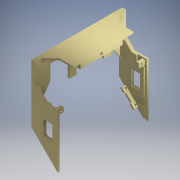
# Autodesk Inventor part: obudowa
Saved by Autodesk Inventor 2017 (Build 210142000, 142)
## iProperties
Created: 2016-11-10
Part Number: obudowa
Material: Generic
Document SubType Name: Modeling
Designer: Shichi
Density: 1 g/cm^3
Appearance: Gold - Metal
Author: Shichi
Autodesk Inventor part; units mm, degrees
ref_plane "YZ Plane" through (0, 0, 0) normal (1, 0, 0) x (0, 1, 0)
ref_plane "XZ Plane" through (0, 0, 0) normal (0, 1, 0) x (-1, 0, 0)
ref_plane "XY Plane" through (0, 0, 0) normal (0, 0, 1) x (1, 0, 0)
sketch "Sketch1" plane through (0, 0, 0) normal (0, 1, 0) x (-1, 0, 0)
  line L0 (0, 0) -> (29, 0)
  line L1 (29, 0) -> (29, 64)
  line L2 (29, 64) -> (25, 64)
  line L3 (25, 64) -> (25, 30)
  line L4 (25, 30) -> (0, 30)
  line L5 (0, 30) -> (0, 0)
  line L6 (29, 0) -> (0, -29)
  line L7 (0, 0) -> (0, -29)
  dimension "d0" = 29
  dimension "d1" = 64
  dimension "d2" = 4
  dimension "d47" = 34
  dimension "d48" = 45
  constraints: 16 end point, 5 perpendicular, 1 horizontal, 1 vertical
  measures "d0" distance of L0.start L0.end
  measures "d1" distance of L0.end L1.end
  measures "d2" distance of L1.end L2.end
  measures "d47" distance of L2.end L3.end
  measures "d48" angle of L6 L0
extrude "Extrusion1" add sketch "Sketch1" along normal blind 2
sketch "Sketch4" plane through (-29, 0, 64) normal (0, 0, 1) x (1, 0, 0)
  line L0 (29, 2) -> (0, 2) projected
  line L1 (0, 2) -> (0, 50)
  line L2 (4, 0) -> (4, 2) projected
  line L3 (4, 2) -> (4, 17)
  line L4 (4, 17) -> (29, 17)
  line L5 (29, 17) -> (29, 50)
  line L6 (0, 50) -> (29, 50)
  point P0 (29, 0)
  dimension "d6" = 48
  dimension "d7" = 15
  dimension "d8" = 25
  dimension "d9" = 33
  constraints: 10 end point, 2 vertical alignment, 1 horizontal, 1 vertical
  measures "d6" distance of L0.end L1.end
  measures "d7" distance of L2.end L3.end
  measures "d8" distance of L3.end L4.end
  measures "d9" distance of L4.end L5.end
extrude "Extrusion2" add sketch "Sketch4" against normal blind 2
ref_plane "Work Plane1" through (0, 50, 0) normal (0, 1, 0) x (1, 0, 0)
mirror "Mirror2" about plane through (0, 50, 0) normal (0, 1, 0) of "Extrusion1"
mirror "Mirror1" about plane through (-29, 50, 64) normal (0, 1, 0) of "Extrusion2"
sketch "Sketch6" plane through (-29, 0, 0) normal (-1, 0, 0) x (0, 0, 1)
  line L0 (62, 17) -> (62, 83) projected
  line L1 (62, 66) -> (16.2993, 98)
  line L2 (62, 98) -> (30, 98) projected
  line L3 (62, 98) -> (62, 66)
  line L4 (16.2993, 98) -> (62, 98)
  point P0 (0, 0)
  dimension "d13" = 32
  dimension "d14" = 55
  constraints: 6 end point, 2 point on line, 1 collinear, 1 vertical
  measures "d13" distance of L2.start L1.start
  measures "d14" angle of L1 L3
extrude "Extrusion3" add sketch "Sketch6" against normal blind 4
sketch "Sketch8" plane through (0, 0, 30) normal (1, 0, 0) x (0, 0, -1)
  line L0 (0, 0) -> (0, 2) projected
  line L1 (0, 2) -> (59, 2) projected
  line L2 (1.5, 2) -> (6.5, 2)
  line L3 (6.5, 2) -> (6.5, 8.5)
  line L4 (6.5, 8.5) -> (1.5, 8.5)
  line L5 (1.5, 8.5) -> (1.5, 2)
  line L6 (-32, 2) -> (0, 2) construction
  line L7 (0, 2) -> (0, 17.9945) construction
  circle A0 centre (4, 6) radius 1.25
  point P0 (30, 0)
  point P1 (30, 2)
  dimension "d17" = 6.5
  dimension "d18" = 6.5
  dimension "d22" = 1.5
  dimension "d23" = 2.5
  dimension "d24" = 4
  dimension "d25" = 4
  constraints: 10 end point, 2 horizontal alignment, 2 parallel, 1 centre point, 1 horizontal, 1 perpendicular, 1 point on line, 1 vertical, 1 vertical alignment
  measures "d17" distance of L4.end L2.start
  measures "d18" distance between parallel lines of L3 L7
  measures "d22" distance between parallel lines of L7 L5
  measures "d23" diameter of A0
  measures "d24" horizontal distance of L0.end A0.centre
  measures "d25" distance from line of A0.centre L1
extrude "Extrusion4" add sketch "Sketch8" against normal blind 5
sketch "Sketch9" plane through (0, 17, 64) normal (1, 0, 0) x (0, 0, -1)
  circle A0 centre (5.7, 33) radius 1.25
  line L0 (2, 0) -> (2, 66) projected
  line L1 (0, 66) -> (2, 66) projected
  line L2 (2, 36.25) -> (8.95, 36.25)
  line L3 (8.95, 36.25) -> (8.95, 29.75)
  line L4 (8.95, 29.75) -> (2, 29.75)
  line L5 (2, 29.75) -> (2, 36.25)
  line L6 (5.7, 34.25) -> (7.6582, 34.25) construction
  line L7 (6.95, 33) -> (6.95, 31.8854) construction
  point P0 (64, -17)
  dimension "d28" = 2.5
  dimension "d29" = 3.7
  dimension "d30" = 33
  dimension "d32" = 2
  dimension "d33" = 4.5
  dimension "d34" = 2
  constraints: 12 end point, 2 horizontal, 2 parallel, 2 point on circle, 2 tangent, 1 centre point, 1 perpendicular, 1 point on line, 1 vertical
  measures "d28" diameter of A0
  measures "d29" distance from line of L0 A0.centre
  measures "d30" distance from line of A0.centre L1
  measures "d32" distance between parallel lines of L2 L6
  measures "d33" distance between parallel lines of L4 L6
  measures "d34" distance between parallel lines of L3 L7
extrude "Extrusion5" add sketch "Sketch9" against normal blind 5
extrude "Extrusion6" cut sketch "Sketch8" against normal blind 2
mirror "Mirror3" about plane through (0, 50, 0) normal (0, 1, 0) of "Extrusion3", "Extrusion4", "Extrusion6"
extrude "Extrusion7" cut sketch "Sketch9" against normal blind 2
sketch "Sketch10" plane through (-29, 0, 62) normal (0, 0, -1) x (-1, 0, 0)
  line L0 (-15, 27) -> (-13, 27)
  line L1 (-13, 27) -> (-13, 35)
  line L2 (-13, 35) -> (-15, 35)
  line L3 (-15, 35) -> (-15, 27)
  line L4 (-24, 53.25) -> (-24, 46.75) projected
  line L5 (-29, 17) -> (-4, 17) projected
  line L6 (-29, 17) -> (-29, 83) construction
  line L7 (-29, 50) -> (0, 50) construction
  line L8 (0, 34) -> (0, 66) construction
  line L9 (-15, 73) -> (-13, 73)
  line L10 (-13, 73) -> (-13, 65)
  line L11 (-13, 65) -> (-15, 65)
  line L12 (-15, 65) -> (-15, 73)
  point P0 (-29, 0)
  point P1 (-15, 31)
  dimension "d41" = 9
  dimension "d42" = 2
  dimension "d43" = 8
  dimension "d46" = 10
  constraints: 18 end point, 4 symmetric about line, 3 midpoint, 2 parallel, 1 horizontal, 1 perpendicular
  measures "d41" distance between parallel lines of L4 L3
  measures "d42" distance of L0.start L0.end
  measures "d43" distance of L0.end L1.end
  measures "d46" distance from line of L5 L0.end
extrude "Extrusion8" add sketch "Sketch10" along normal blind 22
sketch "Sketch11" plane through (-25, 100, 30) normal (0, 1, 0) x (1, 0, 0)
  line L0 (9, 16) -> (19, 16)
  line L1 (19, 16) -> (19, 33)
  line L2 (19, 33) -> (9, 33)
  line L3 (9, 33) -> (9, 16)
  line L4 (0, 0) -> (25, 0) projected
  line L5 (25, 0) -> (25, 59) projected
  point P0 (25, 30)
  dimension "d49" = 16
  dimension "d50" = 6
  dimension "d51" = 10
  dimension "d52" = 17
  constraints: 8 end point, 2 parallel, 1 horizontal, 1 horizontal alignment, 1 perpendicular
  measures "d49" distance between parallel lines of L4 L0
  measures "d50" distance between parallel lines of L5 L1
  measures "d51" distance of L1.end L2.end
  measures "d52" distance of L0.end L1.end
extrude "Extrusion9" cut sketch "Sketch11" against normal through all
sketch "Sketch12" plane through (-29, 0, 0) normal (-0.7071068, 0, -0.7071068) x (-0.7071068, 0, 0.7071068)
  line L0 (0.7071, 2) -> (-41.0122, 2) projected
  line L1 (-8, 2) -> (-13, 2)
  line L2 (-13, 2) -> (-13, 8)
  line L3 (-13, 8) -> (-8, 8)
  line L4 (-8, 8) -> (-8, 2)
  line L5 (-23, 2) -> (-28, 2)
  line L6 (-28, 2) -> (-28, 8)
  line L7 (-28, 8) -> (-23, 8)
  line L8 (-23, 8) -> (-23, 2)
  line L9 (0, 0) -> (0, 2) projected
  circle A0 centre (-10.5, 5) radius 1.25
  circle A1 centre (-25.5, 5) radius 1.25
  point P0 (-20.5061, 0)
  dimension "d55" = 8
  dimension "d56" = 5
  dimension "d57" = 6
  dimension "d58" = 10
  dimension "d59" = 5
  dimension "d60" = 6
  dimension "d61" = 2.5
  dimension "d62" = 2.5
  dimension "d63" = 3
  dimension "d64" = 2.5
  dimension "d65" = 3
  dimension "d66" = 2.5
  constraints: 16 end point, 4 parallel, 2 centre point, 2 horizontal, 2 perpendicular, 2 point on line
  measures "d55" distance between parallel lines of L4 L9
  measures "d56" distance of L2.end L3.end
  measures "d57" distance of L1.end L2.end
  measures "d58" distance between parallel lines of L2 L8
  measures "d59" distance of L6.end L7.end
  measures "d60" distance of L7.end L5.start
  measures "d61" diameter of A0
  measures "d62" distance from line of L4 A0.centre
  measures "d63" distance from line of L0 A0.centre
  measures "d64" distance from line of L8 A1.centre
  measures "d65" distance from line of L0 A1.centre
  measures "d66" diameter of A1
extrude "Extrusion10" add sketch "Sketch12" against normal blind 2
mirror "Mirror4" about plane through (0, 50, 0) normal (0, 1, 0) of "Extrusion10"
sketch "Sketch13" plane through (-25, 98, 30) normal (0, -1, 0) x (1, 0, 0)
  line L0 (-4, -13.7007) -> (0, -13.7007) projected
  line L1 (-4, -13.7007) -> (0, -13.7007)
  line L2 (0, -13.7007) -> (0, 0) projected
  line L3 (25, 0) -> (25, -59) projected
  line L4 (25, -59) -> (-4, -30) projected
  line L5 (15.799, -49.799) -> (17.2132, -48.3848) projected
  line L6 (17.2132, -48.3848) -> (13.6777, -44.8492) projected
  line L7 (13.6777, -44.8492) -> (12.2635, -46.2635) projected
  line L8 (5.1924, -39.1924) -> (6.6066, -37.7782) projected
  line L9 (6.6066, -37.7782) -> (3.0711, -34.2426) projected
  line L10 (3.0711, -34.2426) -> (1.6569, -35.6569) projected
  line L11 (25, -59) -> (15.799, -49.799) projected
  line L12 (17.2132, -48.3848) -> (15.799, -49.799) projected
  line L13 (23, -57) -> (15.799, -49.799)
  line L14 (15.799, -49.799) -> (17.2132, -48.3848)
  line L15 (17.2132, -48.3848) -> (13.6777, -44.8492)
  line L16 (12.2635, -46.2635) -> (13.6777, -44.8492) projected
  line L17 (12.2635, -46.2635) -> (5.1924, -39.1924) projected
  line L18 (12.2635, -46.2635) -> (5.1924, -39.1924)
  line L19 (6.6066, -37.7782) -> (5.1924, -39.1924) projected
  line L20 (5.1924, -39.1924) -> (6.6066, -37.7782)
  line L21 (6.6066, -37.7782) -> (3.0711, -34.2426)
  line L22 (1.6569, -35.6569) -> (-4, -30) projected
  line L23 (1.6569, -35.6569) -> (-4, -30)
  line L24 (-4, -30) -> (-4, -13.7007) projected
  line L25 (-4, -30) -> (-4, -13.7007)
  line L26 (0, -13.7007) -> (0, 0)
  line L27 (0, 0) -> (15, 0)
  line L28 (0, 0) -> (25, 0) projected
  line L29 (15, 0) -> (15, -8)
  line L30 (15, -8) -> (23, -8)
  line L31 (23, -8) -> (23, -57)
  line L32 (9, -33) -> (9, -16) projected
  line L33 (9, -33) -> (19, -33)
  line L34 (9, -16) -> (19, -16) projected
  line L35 (19, -33) -> (19, -16)
  line L36 (19, -16) -> (9, -16)
  line L37 (9, -16) -> (9, -33)
  point P0 (25, -30)
  dimension "d71" = 15
  dimension "d73" = 8
  constraints: 36 end point, 9 collinear, 4 perpendicular, 2 point on line, 2 vertical, 1 horizontal
  measures "d71" distance of L2.end L27.end
  measures "d73" distance of L27.end L29.end
extrude "Extrusion12" add sketch "Sketch13" along normal blind 1.5 contours L0 L2 L27 L29 L30 L31 L4 L5 L6 L7 L8 L9 L10 L24
sketch "Sketch15" plane through (-25, 96.5, 16.2993) normal (-1, 0, 0) x (0, 0, 1)
  line L0 (0, 1.5) -> (45.7007, -30.5) projected
  line L1 (0, 1.5) -> (0, 0) projected
  line L2 (0, 1.5) -> (0, 0) projected
  line L3 (0, 1.5) -> (0, 0)
  line L4 (0, 0) -> (2.1422, 0)
  line L5 (2.1422, 0) -> (0, 0) projected
  line L6 (0, 1.5) -> (0, 0)
  point P0 (-16.2993, -96.5)
  constraints: 6 end point, 2 perpendicular, 1 point on line, 1 vertical
extrude "Extrusion13" add sketch "Sketch15" along normal blind 4
mirror "Mirror5" about plane through (0, 50, 0) normal (0, 1, 0) of "Extrusion12", "Extrusion13"
sketch "Sketch16" plane through (-29, 0, 0) normal (-1, 0, 0) x (0, 0, 1)
  line L0 (64, 100) -> (30, 100) construction
  line L1 (54, 100) -> (54, 55.4894) construction
  line L2 (64, 0) -> (64, 100) construction
  line L3 (64, 83) -> (15.2658, 83) construction
  line L4 (54, 83) -> (37.7215, 83)
  line L5 (62, 66) -> (18.4415, 96.5) projected
  line L6 (37.7215, 83) -> (54, 71.6017)
  line L7 (54, 83) -> (54, 71.6017)
  point P0 (0, 0)
  dimension "d78" = 17
  dimension "d79" = 10
  constraints: 10 end point, 8 point on line, 1 collinear, 1 horizontal, 1 vertical
  measures "d78" distance between parallel lines of L0 L3
  measures "d79" distance between parallel lines of L2 L1
extrude "Extrusion14" cut sketch "Sketch16" against normal blind 4
mirror "Mirror6" about plane through (0, 50, 0) normal (0, 1, 0) of "Extrusion14"
sketch "Sketch17" plane through (-25, 100, 30) normal (0, 1, 0) x (1, 0, 0)
  line L0 (0, 0) -> (0, 11.5585) projected
  line L1 (0, 0) -> (10, 0)
  line L2 (0, 0) -> (25, 0) projected
  line L3 (0, 0) -> (0, -10)
  line L4 (0, -7.7215) -> (0, 11.5585) projected
  line L5 (0, -10) -> (10, 0)
  point P0 (25, 30)
  dimension "d82" = 10
  dimension "d83" = 10
  constraints: 6 end point, 2 point on line
  measures "d82" distance of L0.start L1.end
  measures "d83" distance of L0.start L3.end
extrude "Extrusion15" add sketch "Sketch17" against normal blind 3.5
sketch "Sketch18" plane through (-29, 0, 64) normal (0, 0, 1) x (1, 0, 0)
  line L0 (4, 83) -> (4, 96.5) projected
  line L1 (4, 83) -> (14, 83)
  line L2 (4, 83) -> (29, 83) projected
  line L3 (4, 83) -> (4, 93)
  line L4 (4, 93) -> (14, 83)
  point P0 (29, 0)
  dimension "d86" = 10
  dimension "d87" = 10
  constraints: 6 end point, 2 point on line
  measures "d86" distance of L0.start L1.end
  measures "d87" distance of L0.start L3.end
extrude "Extrusion16" add sketch "Sketch18" against normal blind 2
mirror "Mirror7" about plane through (0, 50, 0) normal (0, 1, 0) of "Extrusion16", "Extrusion15"
sketch "Sketch19" plane through (-29, 0, 0) normal (-1, 0, 0) x (0, 0, 1)
  line L0 (62, 34) -> (62, 66) construction
  line L1 (62, 58.502) -> (62, 57.502) construction
  line L2 (62, 57.502) -> (62, 56.502) construction
  line L3 (62, 40.5076) -> (61, 40.5076) construction
  line L4 (61, 40.5076) -> (61, 33.2998)
  line L5 (54, 28.3983) -> (62, 34) projected
  line L6 (62, 34) -> (62, 66)
  line L7 (62, 66) -> (54, 71.6017) projected
  line L8 (61, 66.7002) -> (61, 40.5076)
  point P0 (0, 0)
  dimension "d92" = 1
  constraints: 12 end point, 7 point on line, 1 collinear, 1 parallel, 1 perpendicular, 1 vertical
  measures "d92" distance of L3.start L3.end
extrude "Extrusion17" add sketch "Sketch19" against normal blind 4
chamfer "Chamfer1" distance 3 angle 45 3 edges at (-25, 96.5, 29.2207) (-25, 50, 62) (-25, 3.5, 29.2207)
sketch "Sketch21" plane through (-2, 17, 64) normal (1, 0, 0) x (0, 0, -1)
  line L0 (2, 36.25) -> (8.95, 36.25) projected
  line L1 (2, 0) -> (2, 66) projected
  line L2 (8.95, 29.75) -> (2, 29.75) projected
  line L3 (2, 36.25) -> (2, 66)
  line L4 (2, 66) -> (0, 66) projected
  line L5 (8.95, 36.25) -> (8.95, 29.75) projected
  line L6 (2, 36.25) -> (8.95, 36.25)
  line L7 (8.95, 36.25) -> (8.95, 56.25)
  line L8 (2, 56) -> (2, 48) projected
  line L9 (8.95, 56.25) -> (2, 56.25)
  line L10 (2, 36.25) -> (2, 56.25)
  point P0 (64, -17)
  dimension "d100" = 20
  constraints: 10 end point, 2 collinear, 2 perpendicular, 1 horizontal, 1 point on line
  measures "d100" distance of L0.end L7.end
extrude "Extrusion18" add sketch "Sketch21" against normal blind 3 contours L1 L9 L7 L0
mirror "Mirror8" about plane through (0, 50, 0) normal (0, 1, 0) of "Extrusion18"
chamfer "Chamfer2" distance 7 angle 45 2 edges at (-14, 69, 62) (-14, 31, 62)
sketch "Sketch22" plane through (0, 98, -29) normal (-0.7071068, 0, -0.7071068) x (-0.7071068, 0, 0.7071068)
  line L0 (28.0122, -94.5) -> (28.0122, -90) projected
  line L1 (28.0122, -94.5) -> (28.0122, -91)
  line L2 (28.0122, -91) -> (18.0122, -91)
  line L3 (18.0122, -94.5) -> (18.0122, -90) projected
  line L4 (18.0122, -94.5) -> (28.0122, -94.5)
  line L5 (34.6482, -94.5) -> (22.6274, -94.5) projected
  point P0 (20.5061, -98)
  dimension "d106" = 3.5
  constraints: 6 end point, 2 point on line, 1 collinear, 1 perpendicular
  measures "d106" distance of L0.start L1.end
extrude "Extrusion19" add sketch "Sketch22" against normal blind 2
mirror "Mirror9" about plane through (0, 50, 0) normal (0, 1, 0) of "Extrusion19"
chamfer "Chamfer5" distance 1 angle 45 4 edges at (-19.1005, 93, -8.4853) (-12.0294, 93, -15.5563) (-19.1005, 7, -8.4853) (-12.0294, 7, -15.5563)
sketch "Sketch23" plane through (-25, 96.5, 30) normal (0, -1, 0) x (1, 0, 0)
  line L0 (25, -59) -> (23, -57) projected
  line L1 (23, -57) -> (23, -8) projected
  line L2 (23, -38) -> (16, -38)
  line L3 (15.799, -49.799) -> (23, -57) projected
  line L4 (16, -38) -> (16, -46)
  line L5 (23, -46) -> (16, -46)
  line L6 (23, -46) -> (23, -38)
  point P0 (25, -30)
  dimension "d118" = 19
  dimension "d119" = 7
  dimension "d120" = 8
  dimension "d121" = 90
  dimension "d122" = 90
  dimension "d123" = 90
  constraints: 8 end point, 2 point on line, 1 collinear
  measures "d118" distance of L0.end L2.start
  measures "d119" distance of L2.start L2.end
  measures "d120" distance of L2.end L4.end
  measures "d121" angle of L1 L5
  measures "d122" angle of L1 L2
  measures "d123" angle of L5 L4
extrude "Extrusion20" cut sketch "Sketch23" against normal blind 1.5
mirror "Mirror10" about plane through (0, 50, 0) normal (0, 1, 0) of "Extrusion20"
body "Solid1"
